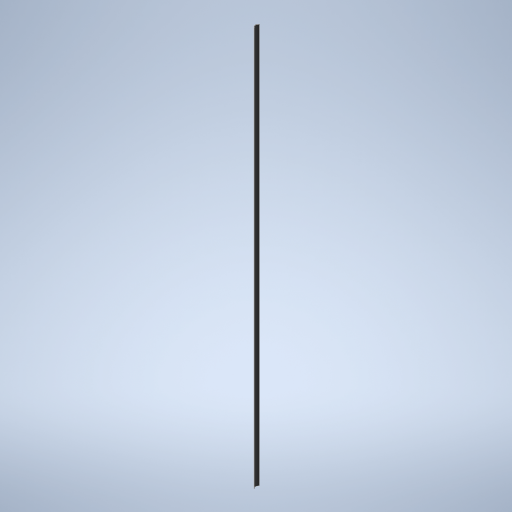
# Autodesk Inventor part: 11.8inch bands
Saved by Autodesk Inventor 2023 (Build 270158000, 158)
## iProperties
Created: 2022-05-22
Part Number: 11.8inch bands
Material: Rubber, Silicone
Document SubType Name: Modeling
Designer: aaron
Density: 1.25 g/cm^3
Appearance: Rubber - Black
Author: aaron
Autodesk Inventor part; units mm, degrees
ref_plane "YZ Plane" through (0, 0, 0) normal (1, 0, 0) x (0, 1, 0)
ref_plane "XZ Plane" through (0, 0, 0) normal (0, 1, 0) x (-1, 0, 0)
ref_plane "XY Plane" through (0, 0, 0) normal (0, 0, 1) x (1, 0, 0)
sketch "Sketch1" plane through (0, 0, 0) normal (0, 1, 0) x (-1, 0, 0)
  circle A0 centre (0, 0) radius 2.54
  line L0 (0, 0) -> (0, 2.54)
  line L1 (0, 0) -> (1.27, 2.1997)
  line L2 (0, 0) -> (2.54, 0) construction
  line L3 (0, 0) -> (1.27, -2.1997)
  line L4 (0, 0) -> (2.54, 0) construction
  circle A1 centre (0, 0) radius 2.1431
  point P0 (1.0716, 1.856)
  point P1 (1.0716, -1.856)
  dimension "d0" = 5.08
  dimension "d1" = 60
  dimension "d2" = 60
  dimension "d3" = 0.3969
  constraints: 10 end point, 3 point on circle, 2 centre point, 2 equal length, 2 horizontal, 1 coincident, 1 vertical
  measures "d0" diameter of A0
  measures "d1" angle of L2 L1
  measures "d2" angle of L3 L4
  measures "d3" radial gap between concentric circles of A0 A1
extrude "Extrusion1" add sketch "Sketch1" along normal blind 299.72 contours A0 L3 A1 L1
fillet "Fillet1" radius 0.1984 4 edges at (-1.0716, 149.86, 1.856) (-1.27, 149.86, 2.1997) (-1.0716, 149.86, -1.856) (-1.27, 149.86, -2.1997)
body "Solid1"
